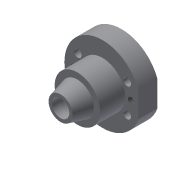
# Autodesk Inventor part: Core
Saved by Autodesk Inventor 2022 (Build 260148000, 148)
## iProperties
Shininess: 64.0
Length Units: 11269
Angle Units: 11279
Time Units: 11290
Mass Units: 11283
Length Display Precision: 3
Angle Display Precision: 2
Compacted: True
Part Number: Core
Document SubType Name: Modeling
Created: 2003-04-04
Designer: demo
Density: 1 g/cm^3
Material: Generic
Appearance: Default
Density: 0.0
Volumn: 0.0
Area: 0.0
PropertySet Name: Model Information
Control State: 0
Master: False
Checked Out: False
Author: demo
Autodesk Inventor part; units mm, degrees
sketch "Sketch1" plane through (0, 0, 0) normal (0, 0, 1) x (1, 0, 0)
  circle A0 centre (-1.4212, 6.3953) radius 31.75
  dimension "d0" = 63.5
  constraints: 1 centre point
  measures "d0" diameter of A0
extrude "Extrusion1" add sketch "Sketch1" along normal blind 15.875
sketch "Sketch2" plane through (-1.4212, 6.3953, 15.875) normal (0, 0, 1) x (1, 0, 0)
  circle A0 centre (0, 0) radius 31.75 projected
  circle A1 centre (0, 0) radius 18.923
  dimension "d3" = 37.846
  constraints: 1 centre point, 1 coincident, 1 concentric
  measures "d3" diameter of A1
extrude "Extrusion2" add sketch "Sketch2" along normal blind 20.9804 contours A1
sketch "Sketch3" plane through (-1.4212, 6.3953, 36.8554) normal (0, 0, 1) x (1, 0, 0)
  circle A0 centre (0, 0) radius 18.923 projected
  circle A1 centre (0, 0) radius 13.7541
  dimension "d6" = 27.5082
  constraints: 1 centre point, 1 coincident, 1 concentric
  measures "d6" diameter of A1
extrude "Extrusion3" add sketch "Sketch3" along normal blind 13.97 draft -15 contours A1
sketch "Sketch5" plane through (-1.4212, 6.3953, 0) normal (0, 0, -1) x (-1, 0, 0)
  circle A0 centre (0, 0) radius 31.75 projected
  circle A1 centre (0, 0) radius 6.096
  dimension "d12" = 12.192
  constraints: 1 centre point, 1 coincident, 1 concentric
  measures "d12" diameter of A1
extrude "Extrusion5" cut sketch "Sketch5" against normal blind 86.2076 contours A1
sketch "Sketch6" plane through (-1.4212, 6.3953, 0) normal (0, 0, -1) x (-1, 0, 0)
  circle A0 centre (0, 0) radius 31.75 projected
  circle A1 centre (0, 0) radius 6.731
  dimension "d15" = 13.462
  constraints: 1 centre point, 1 coincident, 1 concentric
  measures "d15" diameter of A1
extrude "Extrusion6" cut sketch "Sketch6" against normal blind 77.0128 contours A1
sketch "Sketch7" plane through (-1.4212, 6.3953, 0) normal (0, 0, -1) x (-1, 0, 0)
  circle A0 centre (0, 0) radius 31.75 projected
  circle A1 centre (0, 0) radius 7.239
  dimension "d18" = 14.478
  constraints: 1 centre point, 1 coincident, 1 concentric
  measures "d18" diameter of A1
extrude "Extrusion7" cut sketch "Sketch7" against normal blind 66.6242 contours A1
sketch "Sketch8" plane through (-1.4212, 6.3953, 0) normal (0, 0, -1) x (-1, 0, 0)
  circle A0 centre (0, 0) radius 7.239 projected
  circle A1 centre (0, 0) radius 31.75 projected
  circle A2 centre (0, 0) radius 12.192
  dimension "d21" = 24.384
  constraints: 1 centre point, 1 coincident, 1 concentric
  measures "d21" diameter of A2
extrude "Extrusion8" cut sketch "Sketch8" against normal blind 6.35 contours A2
sketch "Sketch9" plane through (-1.4212, 6.3953, 6.35) normal (0, 0, -1) x (-1, 0, 0)
  circle A0 centre (0, 0) radius 7.239 projected
  circle A1 centre (0, 0) radius 12.192 projected
  circle A2 centre (0, 0) radius 9.525
  dimension "d24" = 19.05
  constraints: 1 centre point, 1 coincident, 1 concentric
  measures "d24" diameter of A2
extrude "Extrusion9" cut sketch "Sketch9" against normal blind 24.8158 contours A2
sketch "Sketch10" plane through (-1.4212, 6.3953, 31.1658) normal (0, 0, -1) x (-1, 0, 0)
  circle A0 centre (0, 0) radius 9.525 projected
extrude "Extrusion10" cut sketch "Sketch10" against normal blind 12.954 draft -10
sketch "Sketch11" plane through (-1.4212, 6.3953, 0) normal (0, 0, -1) x (-1, 0, 0)
  circle A0 centre (0, 0) radius 31.75 projected
  line L0 (0, 0) -> (0, 36.2783)
  line L1 (-29.972, -10.4758) -> (-29.972, 10.4758)
  dimension "d29" = 29.972
  constraints: 4 end point, 2 point on circle, 1 vertical
  measures "d29" distance between parallel lines of L0 L1
extrude "Extrusion11" cut sketch "Sketch11" against normal through all contours L1 A0 picked at (-30.4983, 1.1837)
ref_plane "Work Plane1" through (-1.4212, 6.3953, 6.35) normal (0, 1, 0) x (0, 0, 1)
ref_plane "Work Plane2" through (-1.4212, 6.3953, 6.35) normal (1, 0, 0) x (0, 0, 1)
sketch "Sketch12" plane through (0, 0, 0) normal (0, 0, -1) x (-1, 0, 0)
  circle A0 centre (1.4212, 6.3953) radius 12.192 projected
  line L0 (-47.0674, 6.3953) -> (39.3434, 6.3953) projected
  circle A1 centre (1.4212, 6.3953) radius 23.7998
  point P0 (-22.3786, 6.3953)
  point P1 (25.221, 6.3953)
  dimension "d34" = 47.5996
  constraints: 2 point on circle, 2 point on line, 1 centre point, 1 coincident, 1 concentric
  measures "d34" diameter of A1
hole "Hole1" at (22.3786, 6.3953, 0) at (-25.221, 6.3953, 0) direction (0, 0, 1) diameter 4.9784 end through all thread size "1/4-20 UNC" class "1B" standard "ANSI Unified Screw Threads"
sketch "Sketch13" plane through (0, 0, 0) normal (0, 0, -1) x (-1, 0, 0)
  circle A0 centre (1.4212, 6.3953) radius 12.192 projected
  circle A1 centre (1.4212, 6.3953) radius 23.7858
  line L0 (1.4212, 6.3953) -> (23.4182, 19.0953)
  line L1 (1.4212, 6.3953) -> (-20.5759, 19.0953)
  line L2 (1.4212, 6.3953) -> (-20.5759, -6.3047)
  line L3 (1.4212, 6.3953) -> (23.4182, -6.3047)
  point P0 (-19.1779, 18.2883)
  point P1 (22.0203, 18.2883)
  point P2 (22.0203, -5.4976)
  point P3 (-19.1779, -5.4976)
  constraints: 8 end point, 4 point on circle, 4 point on line, 2 collinear, 1 centre point, 1 coincident, 1 concentric
hole "Hole2" at (19.1779, 18.2883, 0) at (-22.0203, 18.2883, 0) at (-22.0203, -5.4976, 0) at (19.1779, -5.4976, 0) direction (0, 0, 1) diameter 6.35 end through all counterbore diameter 7.9375 counterbore depth 13.4366
sketch "Sketch14" plane through (-1.4212, 6.3953, 6.35) normal (1, 0, 0) x (0, 0, 1)
  line L0 (-6.35, -22.313) -> (18.656, -7.8757)
  constraints: 2 end point
ref_plane "Work Plane3" through (-1.4212, 28.7083, 0) normal (0, -0.5, 0.8660254) x (1, 0, 0)
ref_plane "Work Plane4" through (-1.4212, 35.0583, -10.9985) normal (0, -0.5, 0.8660254) x (1, 0, 0)
sketch "Sketch16" plane through (-1.4212, 35.0583, -10.9985) normal (0, -0.5, 0.8660254) x (1, 0, 0)
  circle A0 centre (0, 0) radius 2.3813 projected
extrude "Extrusion12" cut sketch "Sketch16" along normal up to next
mirror "Mirror1" about plane through (-1.4212, 6.3953, 6.35) normal (0, 1, 0) of "Extrusion12"
sketch "Sketch17" plane through (-1.4212, 6.3953, 6.35) normal (1, 0, 0) x (0, 0, 1)
  line L0 (-6.35, -25.0626) -> (-6.35, -19.5634) projected
  line L1 (-6.35, -27.0882) -> (-5.08, -27.0882)
  line L2 (-5.08, -27.0882) -> (-5.08, -29.4504)
  line L3 (-5.08, -29.4504) -> (-6.35, -29.4504)
  line L4 (-6.35, -22.313) -> (-3.5699, -22.313)
  line L5 (-6.35, -27.0882) -> (-6.35, -29.4504)
  constraints: 10 end point, 2 parallel, 1 midpoint, 1 perpendicular
revolve "Revolution1" cut sketch "Sketch17" angle 360 about axis through (-1.4212, 28.7083, 0) along (0, 0, 1)
mirror "Mirror2" about plane through (-1.4212, 6.3953, 6.35) normal (0, 1, 0) of "Revolution1"
body "Solid1"
